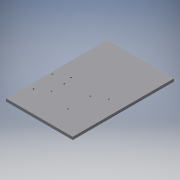
# Autodesk Inventor part: base plate
Saved by Autodesk Inventor 2019 (Build 230136000, 136)
## iProperties
Created: 2019-03-29
Part Number: base plate
Material: Generic
Document SubType Name: Modeling
Designer: Tesler
Density: 1 g/cm^3
Appearance: Default
Author: Tesler
Autodesk Inventor part; units mm, degrees
ref_plane "YZ Plane" through (0, 0, 0) normal (1, 0, 0) x (0, 1, 0)
ref_plane "XZ Plane" through (0, 0, 0) normal (0, 1, 0) x (-1, 0, 0)
ref_plane "XY Plane" through (0, 0, 0) normal (0, 0, 1) x (1, 0, 0)
sketch "Sketch1" plane through (0, 0, 0) normal (0, 1, 0) x (-1, 0, 0)
  line L0 (0, 0) -> (145, 0)
  line L1 (145, 0) -> (145, -220)
  line L2 (145, -220) -> (0, -220)
  line L3 (0, -220) -> (0, 0)
  dimension "d0" = 145
  dimension "d1" = 220
  constraints: 8 end point, 2 parallel, 1 horizontal, 1 perpendicular
  measures "d0" distance of L1.end L2.end
  measures "d1" distance of L0.end L1.end
extrude "Extrusion1" add sketch "Sketch1" along normal blind 6
sketch "Sketch2" plane through (0, 6, 0) normal (0, 1, 0) x (1, 0, 0)
  line L0 (-145, 220) -> (-145, 0) projected
  line L1 (0, 0) -> (0, 220) projected
  line L2 (0, 220) -> (-145, 220) projected
  point P0 (-113.5, 110)
  point P1 (-31.5, 110)
  dimension "d4" = 31.5
  dimension "d5" = 31.5
  dimension "d6" = 110
  dimension "d7" = 110
  measures "d4" distance from line of L0 point (-113.5, 110)
  measures "d5" distance from line of L1 point (-31.5, 110)
  measures "d6" distance from line of L2 point (-113.5, 110)
  measures "d7" distance from line of L2 point (-31.5, 110)
hole "Hole1" at (-113.5, 6, -110) at (-31.5, 6, -110) direction (0, -1, 0) diameter 3 depth 2.5
sketch "Sketch3" plane through (0, 0, 0) normal (0, -1, 0) x (1, 0, 0)
  line L0 (0, 0) -> (-145, 0)
  line L1 (-145, 0) -> (-145, -220)
  line L2 (-145, -220) -> (0, -220)
  line L3 (0, -220) -> (0, 0)
  circle A0 centre (-132.6556, -47.54) radius 1.5621
  circle A1 centre (-109.1479, -62.9815) radius 1.3153
  circle A2 centre (-109.1479, -90.9977) radius 1.5621
  circle A3 centre (-140.1486, -95.8762) radius 1.5621
  circle A4 centre (-57.5224, -95.8762) radius 1.5621
  circle A5 centre (-57.5224, -47.54) radius 1.5621
  circle A6 centre (-132.6556, -47.54) radius 1.5621
  circle A7 centre (-140.1486, -95.8762) radius 1.5621
  circle A8 centre (-109.1479, -90.9977) radius 1.5621
  circle A9 centre (-109.1479, -62.9815) radius 1.3153
  circle A10 centre (-57.5224, -47.54) radius 1.5621
  circle A11 centre (-57.5224, -95.8762) radius 1.5621
extrude "Extrusion2" cut sketch "Sketch3" against normal up to next contours A0 | A1 | A2 | A3 | A4 | A5
equation "\"d5\" = d4"
body "Solid1"
